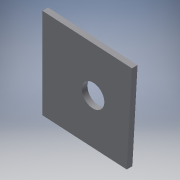
# Autodesk Inventor part: 2018 Intake scissor Plate
Saved by Autodesk Inventor 2018 (Build 220112000, 112)
## iProperties
Created: 2018-01-26
Part Number: 2018 Intake scissor Plate
Material: Generic
Document SubType Name: Modeling
Designer: Apple
Density: 1 g/cm^3
Appearance: Default
Author: Apple
Autodesk Inventor part; units mm, degrees
ref_plane "YZ Plane" through (0, 0, 0) normal (1, 0, 0) x (0, 1, 0)
ref_plane "XZ Plane" through (0, 0, 0) normal (0, 1, 0) x (-1, 0, 0)
ref_plane "XY Plane" through (0, 0, 0) normal (0, 0, 1) x (1, 0, 0)
sketch "Sketch1" plane through (0, 0, 0) normal (0, 0, 1) x (1, 0, 0)
  circle A0 centre (56.8849, 594.6675) radius 12.7 projected
  line L0 (0, 0) -> (0, 736.6) projected
  line L1 (0, 547.0493) -> (94.7709, 541.609)
  line L2 (94.7709, 541.609) -> (100.5936, 643.0421)
  line L3 (100.5936, 643.0421) -> (0, 648.8165)
  line L4 (0, 547.0493) -> (0, 648.8165)
  dimension "d0" = 50.8
  dimension "d1" = 50.8
  constraints: 8 end point, 2 perpendicular, 2 point on line, 1 collinear
  measures "d0" distance from line of L1 A0.centre
  measures "d1" distance from line of L3 A0.centre
extrude "Extrusion1" add sketch "Sketch1" along normal blind 6.35
sketch "Sketch2" plane through (0, 0, 6.35) normal (0, 0, 1) x (1, 0, 0)
  circle A0 centre (12.3052, 635.3893) radius 3.175
  circle A1 centre (12.786, 559.0362) radius 3.175
  line L0 (0, 547.0493) -> (94.7709, 541.609) projected
  line L1 (100.5936, 643.0421) -> (0, 648.8165) projected
  point P0 (0, 0)
  dimension "d4" = 6.35
  dimension "d5" = 6.35
  dimension "d6" = 12.7
  dimension "d7" = 12.7
  constraints: 2 centre point
  measures "d4" diameter of A0
  measures "d5" diameter of A1
  measures "d6" distance from line of A1.centre L0
  measures "d7" distance from line of L1 A0.centre
extrude "Extrusion2" cut sketch "Sketch2" against normal through all
body "Solid1"
